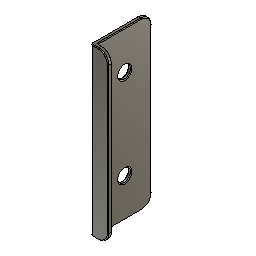
Goalpost (Autodesk Fusion 360 design; units mm, degrees)
Autodesk Fusion 360 part; units mm, degrees
note: some values were not read from the file. Set by a fixed rule: which sketch regions a step uses.
sketch "Skizze1" plane through (0, 0, 0) normal (0, 1, 0) x (1, 0, 0)
  line L0 (0, 0) -> (7, 0)
  line L1 (7, 0) -> (7, -65)
  line L2 (7, -65) -> (0, -65)
  line L3 (0, -65) -> (0, 0)
  dimension "d1" = 7
  dimension "d2" = 65
  constraint horizontal L0
  constraint vertical L1
  constraint horizontal L2
  constraint vertical L3
  constraint coincident L0.start L3.end
  measures "d1" distance of L0.start L0.end
  measures "d2" distance of L0.start L2.end
extrude "Extrusion1" add sketch "Skizze1" along normal blind 1.5
sketch "Skizze2" plane through (0, 1.5, 0) normal (0, 1, 0) x (-1, 0, 0)
  line L0 (0, 65) -> (-7, 65)
  line L1 (-7, 65) -> (-7, 0)
  line L2 (-7, 0) -> (0, 0)
  line L3 (0, 0) -> (0, 65)
  line L4 (-1.5, 65) -> (-1.5, 0)
  dimension "d5" = 1.5
  constraint coincident L0 L4.start
  constraint coincident L2 L4.end
  constraint perpendicular L2 L4
  measures "d5" distance of L3 L4
extrude "Extrusion2" add sketch "Skizze2" along normal blind 21 contours L0 L2 L3 L4
fillet "Abrundung1" radius 4 4 edges at (0.75, 22.5, 65) (7, 0.75, 65) (0.75, 22.5, 0) (7, 0.75, 0)
sketch "Skizze3" plane through (1.5, 0, 0) normal (1, 0, 0) x (0, 1, 0)
  arc A0 (18.5, 0) -> (22.5, 4) centre (18.5, 4) ccw
  line L0 (22.5, 4) -> (22.5, 61)
  arc A1 (22.5, 61) -> (18.5, 65) centre (18.5, 61) ccw
  line L1 (18.5, 65) -> (1.5, 65)
  line L2 (1.5, 65) -> (1.5, 0)
  line L3 (1.5, 0) -> (18.5, 0)
  line L4 (12, 65) -> (12, 0)
  circle A2 centre (12, 50) radius 2.5
  circle A3 centre (12, 15) radius 2.5
  dimension "d10" = 12
  dimension "d11" = 5
  dimension "d12" = 5
  dimension "d13" = 15
  dimension "d14" = 15
  constraint coincident L1 L4.start
  constraint coincident L3 L4.end
  constraint perpendicular L3 L4
  constraint coincident L4 A2.centre
  constraint coincident L4 A3.centre
  measures "d10" distance of origin L4
  measures "d11" diameter of A2
  measures "d12" diameter of A3
  measures "d13" distance of L4.end A3.centre
  measures "d14" distance of L4.start A2.centre
extrude "Extrusion3" cut sketch "Skizze3" against normal blind 2 contours L4 A3 | L4 A3 | L4 A2 | L4 A2
chamfer "Fase1" distance 0.5 angle 45 2 edges at (0, 9.6692, 49.096) (0, 9.6692, 14.096)
fillet "Abrundung4" radius 0.4 1 edges at (1.5, 1.5, 32.5)
fillet "Abrundung6" radius 1 1 edges at (0, 0, 32.5)
fillet "Abrundung7" radius 0.3 26 edges at (1.5, 22.5, 32.5) (1.5, 21.3284, 1.1716) (1.5, 10.2, 0) (1.6172, 1.6172, 0) (2.45, 1.5, 0) (5.8284, 1.5, 1.1716) (7, 1.5, 32.5) (5.8284, 1.5, 63.8284) (2.45, 1.5, 65) (1.6172, 1.6172, 65) (1.5, 10.2, 65) (1.5, 21.3284, 63.8284) (0, 21.3284, 63.8284) (0, 9.75, 65) (0.2929, 0.2929, 65) (2, 0, 65) (5.8284, 0, 63.8284) (7, 0, 32.5) (5.8284, 0, 1.1716) (2, 0, 0) (0.2929, 0.2929, 0) (0, 9.75, 0) (0, 21.3284, 1.1716) (0, 22.5, 32.5) (1.5, 9.6692, 50.904) (1.5, 9.6692, 15.904)
